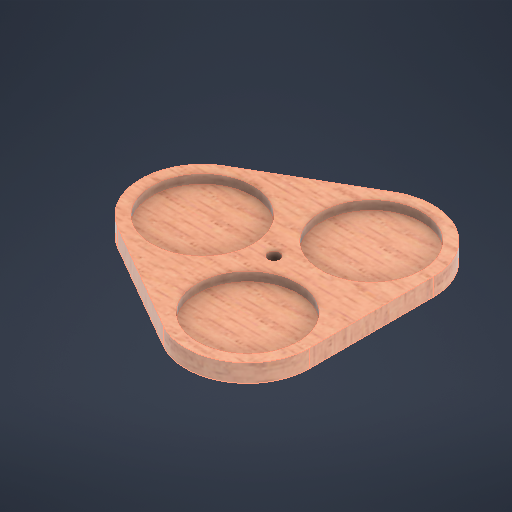
# Autodesk Inventor part: BOTTOM_PLATE_WEIGHTS_TREBUCHET
Saved by Autodesk Inventor 2026.2 (Build 302298010, 298A)
## iProperties
Created: 2026-02-19
Part Number: BOTTOM_PLATE_WEIGHTS_TREBUCHET
Material: Wood (Oak)
Document SubType Name: Modeling
Designer: 4aida
Density: 0.76 g/cm^3
Appearance: White Oak - Natural Medium Gloss
Author: 4aida
Autodesk Inventor part; units mm, degrees
ref_plane "YZ Plane" through (0, 0, 0) normal (1, 0, 0) x (0, 1, 0)
ref_plane "XZ Plane" through (0, 0, 0) normal (0, 1, 0) x (-1, 0, 0)
ref_plane "XY Plane" through (0, 0, 0) normal (0, 0, 1) x (1, 0, 0)
sketch "Sketch1" plane through (0, 0, 0) normal (0, 1, 0) x (-1, 0, 0)
  line L0 (54.6051, -28.5788) -> (-2.5526, -61.5788)
  line L1 (-52.0526, -33) -> (-52.0526, 33)
  line L2 (-2.5526, 61.5788) -> (54.6051, 28.5788)
  circle A0 centre (38.1051, 0) radius 33 construction
  circle A1 centre (-19.0526, 33) radius 33 construction
  circle A2 centre (-19.0526, -33) radius 33 construction
  arc A3 (54.6051, -28.5788) -> (54.6051, 28.5788) centre (38.1051, 0) ccw
  arc A4 (-52.0526, -33) -> (-2.5526, -61.5788) centre (-19.0526, -33) ccw
  arc A5 (-2.5526, 61.5788) -> (-52.0526, 33) centre (-19.0526, 33) ccw
  circle A6 centre (0, 0) radius 3.175
  point P0 (-52.0526, 0)
  dimension "d1" = 66
  dimension "d14" = 6.35
  constraints: 12 point on circle, 9 tangent, 7 centre point, 6 end point, 4 concentric, 2 coincident, 1 horizontal alignment, 1 midpoint, 1 vertical, 4 other
  measures "d1" diameter of A0
  measures "d14" diameter of A6
extrude "Extrusion1" add sketch "Sketch1" along normal blind 9.525
sketch "Sketch2" plane through (0, 9.525, 0) normal (0, 1, 0) x (1, 0, 0)
  circle A0 centre (19.0526, -33) radius 27
  circle A1 centre (-38.1051, 0) radius 27
  circle A2 centre (19.0526, 33) radius 27
  circle A3 centre (19.0526, 33) radius 33
  circle A4 centre (-38.1051, 0) radius 33
  circle A5 centre (19.0526, -33) radius 33
  line L0 (-54.6051, -28.5788) -> (2.5526, -61.5788) projected
  line L1 (2.5526, 61.5788) -> (-54.6051, 28.5788) projected
  line L2 (52.0526, -33) -> (52.0526, 33) projected
  point P0 (0, 0)
  point P1 (-99.3426, -2.7496)
  point P2 (47.2901, -87.408)
  point P3 (47.2901, 87.408)
  point P4 (-99.3426, 2.7496)
  point P5 (52.0526, -84.6584)
  point P6 (52.0526, 84.6584)
  dimension "d5" = 54
  constraints: 9 tangent, 6 centre point, 3 coincident, 2 equal radius
  measures "d5" diameter of A0
extrude "Extrusion2" cut sketch "Sketch2" against normal blind 5 contours A0 | A1 | A2
body "Solid1"
